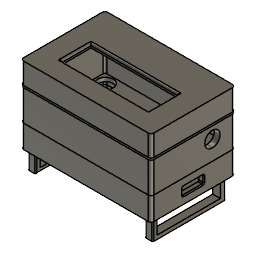
Irfan Hazlan - Device Case CAD Model (Autodesk Fusion 360 archive; units mm, degrees)
design "Irfan Hazlan - Device Case CAD Model" references "Prototype"
part number: 2026-02-20-13-36-55-425
Autodesk Fusion 360 part; units mm, degrees
derive "Sketch1"
sketch "sketch 219" plane through (0, 0, 0) normal (0, 0, 1) x (1, 0, 0)
  line L0 (1.5, 0) -> (66.5, 0)
  line L1 (68, 1.5) -> (68, 42.5)
  line L2 (66.5, 44) -> (1.5, 44)
  line L3 (0, 42.5) -> (0, 1.5)
  arc A0 (1.5, 44) -> (0, 42.5) centre (1.5, 42.5) ccw
  arc A1 (68, 42.5) -> (66.5, 44) centre (66.5, 42.5) ccw
  arc A2 (66.5, 0) -> (68, 1.5) centre (66.5, 1.5) ccw
  arc A3 (0, 1.5) -> (1.5, 0) centre (1.5, 1.5) ccw
  line L4 (2, 41) -> (2, 3)
  line L5 (3, 2) -> (65, 2)
  line L6 (66, 3) -> (66, 41)
  line L7 (65, 42) -> (3, 42)
  line L8 (4, 3) -> (64, 3)
  line L9 (65, 4) -> (65, 40)
  line L10 (64, 41) -> (4, 41)
  line L11 (3, 40) -> (3, 4)
  arc A4 (3, 42) -> (2, 41) centre (3, 41) ccw
  arc A5 (2, 3) -> (3, 2) centre (3, 3) ccw
  arc A6 (65, 2) -> (66, 3) centre (65, 3) ccw
  arc A7 (66, 41) -> (65, 42) centre (65, 41) ccw
  arc A8 (65, 40) -> (64, 41) centre (64, 40) ccw
  arc A9 (4, 41) -> (3, 40) centre (4, 40) ccw
  arc A10 (3, 4) -> (4, 3) centre (4, 4) ccw
  arc A11 (64, 3) -> (65, 4) centre (64, 4) ccw
  arc A12 (164, 3) -> (165, 4) centre (164, 4) ccw
  arc A13 (101.5, 44) -> (100, 42.5) centre (101.5, 42.5) ccw
  arc A14 (100, 1.5) -> (101.5, 0) centre (101.5, 1.5) ccw
  arc A15 (165, 2) -> (166, 3) centre (165, 3) ccw
  line L12 (166, 3) -> (166, 41)
  line L13 (103, 40) -> (103, 4)
  line L14 (165, 42) -> (103, 42)
  line L15 (103, 2) -> (165, 2)
  arc A16 (102, 3) -> (103, 2) centre (103, 3) ccw
  arc A17 (166.5, 0) -> (168, 1.5) centre (166.5, 1.5) ccw
  arc A18 (165, 40) -> (164, 41) centre (164, 40) ccw
  arc A19 (103, 42) -> (102, 41) centre (103, 41) ccw
  arc A20 (166, 41) -> (165, 42) centre (165, 41) ccw
  line L16 (166.5, 44) -> (101.5, 44)
  line L17 (101.5, 0) -> (166.5, 0)
  line L18 (168, 1.5) -> (168, 42.5)
  line L19 (102, 41) -> (102, 3)
  arc A21 (168, 42.5) -> (166.5, 44) centre (166.5, 42.5) ccw
  line L20 (100, 42.5) -> (100, 1.5)
  line L21 (104, 3) -> (164, 3)
  arc A22 (103, 4) -> (104, 3) centre (104, 4) ccw
  line L22 (165, 4) -> (165, 40)
  arc A23 (104, 41) -> (103, 40) centre (104, 40) ccw
  line L23 (164, 41) -> (104, 41)
  arc A24 (264, 3) -> (265, 4) centre (264, 4) ccw
  arc A25 (201.5, 44) -> (200, 42.5) centre (201.5, 42.5) ccw
  arc A26 (200, 1.5) -> (201.5, 0) centre (201.5, 1.5) ccw
  arc A27 (265, 2) -> (266, 3) centre (265, 3) ccw
  line L24 (266, 3) -> (266, 41)
  line L25 (203, 40) -> (203, 4)
  line L26 (265, 42) -> (203, 42)
  line L27 (203, 2) -> (265, 2)
  arc A28 (202, 3) -> (203, 2) centre (203, 3) ccw
  arc A29 (266.5, 0) -> (268, 1.5) centre (266.5, 1.5) ccw
  arc A30 (265, 40) -> (264, 41) centre (264, 40) ccw
  arc A31 (203, 42) -> (202, 41) centre (203, 41) ccw
  arc A32 (266, 41) -> (265, 42) centre (265, 41) ccw
  line L28 (266.5, 44) -> (201.5, 44)
  line L29 (201.5, 0) -> (266.5, 0)
  line L30 (268, 1.5) -> (268, 42.5)
  line L31 (202, 41) -> (202, 3)
  arc A33 (268, 42.5) -> (266.5, 44) centre (266.5, 42.5) ccw
  line L32 (200, 42.5) -> (200, 1.5)
  line L33 (204, 3) -> (264, 3)
  arc A34 (203, 4) -> (204, 3) centre (204, 4) ccw
  line L34 (265, 4) -> (265, 40)
  arc A35 (204, 41) -> (203, 40) centre (204, 40) ccw
  line L35 (264, 41) -> (204, 41)
  point P0 (68, 0)
  point P1 (0, 44)
  point P2 (100, 44)
  point P3 (168, 0)
  point P4 (100, 0)
  point P5 (100, 0)
  point P6 (200, 44)
  point P7 (268, 0)
  point P8 (200, 0)
  point P9 (200, 0)
extrude "Extrude1" add sketch "sketch 219" along normal blind 2 contours L8 L9 L10 L11 A8 A9 A10 A11 makes body 1
extrude "Extrude2" add sketch "sketch 219" along normal blind 10 contours L4 L5 L6 L7 A4 A5 A6 A7 bodies 1
extrude "Extrude3" add sketch "sketch 219" along normal blind 12 contours L0 L1 L2 L3 A0 A1 A2 A3 bodies 1
extrude "Extrude4" add sketch "sketch 219" along normal blind 20 separate body contours A15 L12 L14 L15 A16 A19 A20 L19 makes body 2
extrude "Extrude5" add sketch "sketch 219" along normal blind 2 from surface at 10 contours A12 L13 A18 L21 A22 L22 A23 L23 bodies 2
extrude "Extrude6" add sketch "sketch 219" along normal blind 16 from surface at 2 contours A13 A14 A17 L16 L17 L18 A21 L20 bodies 2
move_face "MoveFace1" by (0, 0, -6) 1 faces at (144, 28.3333, 12) on bodies 2
extrude "Extrude7" add sketch "sketch 219" along normal blind 12 contours A12 L13 A18 L21 A22 L22 A23 L23 bodies 2
sketch "Sketch1" plane through (0, 0, 12) normal (0, 0, 1) x (-1, 0, 0)
  line L0 (-164, -41) -> (-104, -41)
  arc A0 (-104, -41) -> (-103, -40) centre (-104, -40) ccw
  line L1 (-103, -40) -> (-103, -4)
  arc A1 (-103, -4) -> (-104, -3) centre (-104, -4) ccw
  line L2 (-104, -3) -> (-164, -3)
  arc A2 (-164, -3) -> (-165, -4) centre (-164, -4) ccw
  line L3 (-165, -4) -> (-165, -40)
  arc A3 (-165, -40) -> (-164, -41) centre (-164, -40) ccw
  circle A4 centre (-108.0439, -36.228) radius 2.5
  circle A5 centre (-108.0439, -36.228) radius 4
  dimension "d17" = 5
  dimension "d114" = 8
  constraint concentric A4 A5
  measures "d17" diameter of A4
  measures "d114" diameter of A5
extrude "Extrude8" cut sketch "Sketch1" against normal blind 2 contours A4 bodies 2
copy_body "CopyPasteBodies3" bodies 1 makes body 3
move_body "Move2" bodies 3 to x (1, 0, 0) y (0, 1, 0) z (0, 0, 1) at (200, 0, 0)
move_body "Move3" bodies 3 to x (1, 0, 0) y (0, 1, 0) z (0, 0, 1) at (0, 0, 10)
move_body "Move4" bodies 3 to x (-1, 0, 0) y (0, 1, 0) z (0, 0, -1) at (536, 0, 20)
move_body "Move5" bodies 3 to x (1, 0, 0) y (0, 1, 0) z (0, 0, 1) at (-70, 0, 0)
sketch "Sketch2" plane through (0, 0, 10) normal (0, 0, 1) x (-1, 0, 0)
  arc A0 (-264.5, 0) -> (-266, -1.5) centre (-264.5, -1.5) ccw
  line L0 (-266, -1.5) -> (-266, -42.5)
  arc A1 (-266, -42.5) -> (-264.5, -44) centre (-264.5, -42.5) ccw
  line L1 (-264.5, -44) -> (-199.5, -44)
  arc A2 (-199.5, -44) -> (-198, -42.5) centre (-199.5, -42.5) ccw
  line L2 (-198, -42.5) -> (-198, -1.5)
  arc A3 (-198, -1.5) -> (-199.5, 0) centre (-199.5, -1.5) ccw
  line L3 (-199.5, 0) -> (-264.5, 0)
  line L4 (-209.1663, -25.5187) -> (-254.1663, -25.5187)
  line L5 (-254.1663, -25.5187) -> (-254.1663, -10.5187)
  line L6 (-254.1663, -10.5187) -> (-209.1663, -10.5187)
  line L7 (-209.1663, -10.5187) -> (-209.1663, -25.5187)
  dimension "d30" = 45
  dimension "d31" = 15
  constraint horizontal L4
  constraint vertical L5
  constraint horizontal L6
  constraint vertical L7
  measures "d30" distance of L4.start L4.end
  measures "d31" distance of L4.end L5.end
extrude "Extrude9" cut sketch "Sketch2" against normal blind 2 contours L4 L5 L6 L7 bodies 3
fillet "Fillet1" radius 1 2 edges at (254.1663, 18.0187, 10) (231.6663, 25.5187, 10) on bodies 3
fillet "Fillet2" radius 1 2 edges at (232.1663, 10.5187, 10) (209.1663, 18.5187, 10) on bodies 3
sketch "Sketch3" plane through (0, 0, 0) normal (0, 0, -1) x (1, 0, 0)
  arc A0 (1.5, 0) -> (0, -1.5) centre (1.5, -1.5) ccw
  line L0 (0, -1.5) -> (0, -42.5)
  arc A1 (0, -42.5) -> (1.5, -44) centre (1.5, -42.5) ccw
  line L1 (1.5, -44) -> (66.5, -44)
  arc A2 (66.5, -44) -> (68, -42.5) centre (66.5, -42.5) ccw
  line L2 (68, -42.5) -> (68, -1.5)
  arc A3 (68, -1.5) -> (66.5, 0) centre (66.5, -1.5) ccw
  line L3 (66.5, 0) -> (1.5, 0)
  line L4 (66.9452, -39.9907) -> (62.9452, -39.9907)
  line L5 (62.9452, -39.9907) -> (62.9452, -1.9907)
  line L6 (62.9452, -1.9907) -> (66.9452, -1.9907)
  line L7 (66.9452, -1.9907) -> (66.9452, -39.9907)
  line L8 (5.9452, -1.9907) -> (5.9452, -39.9907)
  line L9 (5.9452, -39.9907) -> (1.9452, -39.9907)
  line L10 (1.9452, -39.9907) -> (1.9452, -1.9907)
  line L11 (1.9452, -1.9907) -> (5.9452, -1.9907)
  dimension "d38" = 38
  dimension "d39" = 4
  dimension "d40" = 38
  dimension "d41" = 4
  constraint horizontal L4
  constraint vertical L5
  constraint horizontal L6
  constraint vertical L7
  constraint horizontal L9
  constraint vertical L10
  constraint horizontal L11
  constraint vertical L8
  measures "d38" distance of L4.end L5.end
  measures "d39" distance of L4.start L4.end
  measures "d40" distance of L10.end L9.end
  measures "d41" distance of L8.end L9.end
extrude "Extrude10" add sketch "Sketch3" along normal blind 10 contours L4 L5 L6 L7 bodies 1
extrude "Extrude11" add sketch "Sketch3" along normal blind 10 contours L8 L9 L10 L11 bodies 1
sketch "Sketch4" plane through (1.9452, 0, 0) normal (-1, 0, 0) x (0, -1, 0)
  line L0 (-1.9907, 0) -> (-39.9907, 0)
  line L1 (-39.9907, 0) -> (-39.9907, -10)
  line L2 (-39.9907, -10) -> (-1.9907, -10)
  line L3 (-1.9907, -10) -> (-1.9907, 0)
  line L4 (-37.2414, 0.0076) -> (-4.2414, 0.0076)
  line L5 (-4.2414, 0.0076) -> (-4.2414, -7.9924)
  line L6 (-4.2414, -7.9924) -> (-37.2414, -7.9924)
  line L7 (-37.2414, -7.9924) -> (-37.2414, 0.0076)
  line L8 (-37.2414, -7.9924, -61) -> (-37.2414, 0.0076, -61)
  line L9 (-4.2414, -7.9924, -61) -> (-37.2414, -7.9924, -61)
  line L10 (-4.2414, 0.0076, -61) -> (-4.2414, -7.9924, -61)
  line L11 (-37.2414, 0.0076, -61) -> (-4.2414, 0.0076, -61)
  dimension "d46" = 8
  dimension "d47" = 33
  dimension "d49" = 33
  constraint horizontal L4
  constraint vertical L5
  constraint horizontal L6
  constraint vertical L7
  measures "d46" distance of L4.start L6.end
  measures "d47" distance of L4.start L4.end
  measures "d49" distance of L4.start L4.end
extrude "Extrude12" cut sketch "Sketch4" against normal blind 4 contours L8 L9 L10 L11 in plane through (62.9452, 0, 0) normal (-1, 0, 0) bodies 1
extrude "Extrude13" cut sketch "Sketch4" against normal blind 4 contours L0 L5 L6 L7 | L0 L4 L5 L7 bodies 1
sketch "Sketch5" plane through (0, 2, 0) normal (0, -1, 0) x (1, 0, 0)
  line L0 (165, 2) -> (103, 2)
  line L1 (103, 2) -> (103, 0)
  line L2 (103, 0) -> (165, 0)
  line L3 (165, 0) -> (165, 2)
  line L4 (103, 1) -> (134, 1)
  line L5 (103, 2) -> (134, 0)
  line L6 (103, 0) -> (134, 2)
  line L7 (121, 0.375) -> (116, 0.375)
  line L8 (116, 0.375) -> (116, 1.625)
  line L9 (116, 1.625) -> (121, 1.625)
  line L10 (121, 1.625) -> (121, 0.375)
  line L11 (121, 0.375) -> (116, 1.625) construction
  line L12 (116, 0.375) -> (121, 1.625) construction
  line L13 (134, 2) -> (134, 0)
  line L14 (152, 0.375) -> (152, 1.625)
  line L15 (152, 1.625) -> (147, 1.625)
  line L16 (147, 0.375) -> (152, 0.375)
  line L17 (147, 1.625) -> (147, 0.375)
  point P0 (118.5, 1)
  dimension "d54" = 31
  dimension "d55" = 5
  dimension "d56" = 1.25
  constraint midpoint L1 L4.start
  constraint perpendicular L1 L4
  constraint coincident L0.end L1.start
  constraint midpoint L2 L5.end
  constraint coincident L1.end L2.start
  constraint midpoint L0 L6.end
  constraint horizontal L7
  constraint perpendicular L7 L8
  constraint parallel L7 L9
  constraint parallel L8 L10
  constraint coincident L11 P0
  constraint coincident L12 P0
  constraint midpoint L5 P0
  constraint symmetric L7.start L13 L16.start
  constraint symmetric L7.end L13 L14.start
  constraint symmetric L8.end L13 L14.end
  constraint symmetric L9.end L13 L15.end
  measures "d54" distance of L4.start L4.end
  measures "d55" distance of L8.end L9.end
  measures "d56" distance of L7.end L8.end
sketch "Sketch6" plane through (0, 2, 0) normal (0, -1, 0) x (1, 0, 0)
sketch "Sketch7" plane through (0, 42, 0) normal (0, 1, 0) x (-1, 0, 0)
  line L0 (-103, 2) -> (-165, 2)
  line L1 (-165, 2) -> (-165, 0)
  line L2 (-165, 0) -> (-103, 0)
  line L3 (-103, 0) -> (-103, 2)
  line L4 (-147, 0.375) -> (-152, 0.375)
  line L5 (-147, 1.625) -> (-147, 0.375)
  line L6 (-152, 1.625) -> (-147, 1.625)
  line L7 (-152, 0.375) -> (-152, 1.625)
  line L8 (-116, 1.625) -> (-121, 1.625)
  line L9 (-121, 0.375) -> (-116, 0.375)
  line L10 (-116, 0.375) -> (-116, 1.625)
  line L11 (-121, 1.625) -> (-121, 0.375)
sketch "Sketch8" plane through (0, 0, -2) normal (0, 0, -1) x (1, 0, 0)
  arc A0 (200, -41) -> (201, -42) centre (201, -41) ccw
  line L0 (200, -41) -> (200, -3)
  arc A1 (201, -2) -> (200, -3) centre (201, -3) ccw
  line L1 (201, -2) -> (263, -2)
  arc A2 (264, -3) -> (263, -2) centre (263, -3) ccw
  line L2 (264, -3) -> (264, -41)
  arc A3 (263, -42) -> (264, -41) centre (263, -41) ccw
  line L3 (263, -42) -> (201, -42)
  arc A4 (266, -1.5) -> (264.5, 0) centre (264.5, -1.5) ccw
  line L4 (264.5, 0) -> (199.5, 0)
  arc A5 (199.5, 0) -> (198, -1.5) centre (199.5, -1.5) ccw
  line L5 (198, -1.5) -> (198, -42.5)
  arc A6 (198, -42.5) -> (199.5, -44) centre (199.5, -42.5) ccw
  line L6 (199.5, -44) -> (264.5, -44)
  arc A7 (264.5, -44) -> (266, -42.5) centre (264.5, -42.5) ccw
  line L7 (266, -42.5) -> (266, -1.5)
extrude "Extrude14" add sketch "Sketch7" along normal blind 1 draft -50 contours L4 L5 L6 L7 | L8 L9 L10 L11 bodies 2
extrude "Extrude15" add sketch "Sketch5" along normal blind 1 draft -50 contours L14 L15 L16 L17 bodies 2
extrude "Extrude16" add sketch "Sketch5" along normal blind 1 draft -50 contours L4 L6 L10 | L5 L6 L8 L9 L10 | L4 L5 L8 | L4 L6 L8 | L4 L5 L10 | L5 L6 L7 L8 L10 bodies 2
sketch "Sketch12" plane through (0, 0, 0) normal (0, -1, 0) x (1, 0, 0)
  line L0 (101.5, 2) -> (166.5, 2)
  line L1 (166.5, 2) -> (166.5, 18)
  line L2 (166.5, 18) -> (101.5, 18)
  line L3 (101.5, 18) -> (101.5, 2)
  line L4 (105.009, 18) -> (105.009, 9)
  line L5 (101.5, 9.1208) -> (166.5, 9.1208)
  dimension "d66" = 9
  dimension "d67" = 65
  constraint coincident L2 L4.start
  constraint perpendicular L2 L4
  constraint coincident L3 L5.start
  constraint perpendicular L3 L5
  measures "d66" distance of L4.start L4.end
  measures "d67" distance of L5.start L5.end
sketch "Sketch13" plane through (0, 2, 0) normal (0, -1, 0) x (1, 0, 0)
  line L0 (103, 18) -> (165, 18)
  line L1 (165, 18) -> (165, 20)
  line L2 (165, 20) -> (103, 20)
  line L3 (103, 20) -> (103, 18)
  line L4 (116, 1.625) -> (121, 1.625)
  line L5 (116, 0.375) -> (116, 1.625)
  line L6 (121, 0.375) -> (116, 0.375)
  line L7 (121, 1.625) -> (121, 0.375)
  line L8 (152, 1.625) -> (147, 1.625)
  line L9 (147, 1.625) -> (147, 0.375)
  line L10 (147, 0.375) -> (152, 0.375)
  line L11 (152, 0.375) -> (152, 1.625)
sketch "Sketch14" plane through (0, 2, 0) normal (0, -1, 0) x (1, 0, 0)
  line L0 (134.0523, 17.9964) -> (134.0523, 19.9964)
  line L1 (103.1583, 20.0029) -> (134.0523, 17.9964)
  line L2 (103.1583, 17.9964) -> (134.2435, 20.0029)
  line L3 (121.1529, 18.3716) -> (116.1529, 18.3716)
  line L4 (116.1529, 18.3716) -> (116.1529, 19.6216)
  line L5 (116.1529, 19.6216) -> (121.1529, 19.6216)
  line L6 (121.1529, 19.6216) -> (121.1529, 18.3716)
  line L7 (121.1529, 18.3716) -> (116.1529, 19.6216) construction
  line L8 (116.1529, 18.3716) -> (121.1529, 19.6216) construction
  line L9 (151.9517, 19.6216) -> (146.9517, 19.6216)
  line L10 (151.9517, 18.3716) -> (151.9517, 19.6216)
  line L11 (146.9517, 18.3716) -> (151.9517, 18.3716)
  line L12 (146.9517, 19.6216) -> (146.9517, 18.3716)
  point P0 (118.6529, 18.9966)
  dimension "d68" = 2
  dimension "d69" = 5
  dimension "d70" = 1.25
  constraint vertical L0
  constraint horizontal L3
  constraint perpendicular L3 L4
  constraint parallel L3 L5
  constraint parallel L4 L6
  constraint coincident L7 P0
  constraint coincident L8 P0
  constraint coincident L1 P0
  constraint coincident L2 P0
  constraint symmetric L0 L3.start L11.start
  constraint symmetric L0 L3.end L10.start
  constraint symmetric L0 L4.end L9.start
  constraint symmetric L0 L5.end L9.end
  measures "d68" distance of L0.start L0.end
  measures "d69" distance of L4.end L5.end
  measures "d70" distance of L3.end L4.end
sketch "Sketch15" plane through (0, 2, 0) normal (0, -1, 0) x (1, 0, 0)
  line L0 (116.1529, 19.6216) -> (121.1529, 19.6216)
  line L1 (116.1529, 18.3716) -> (116.1529, 19.6216)
  line L2 (121.1529, 18.3716) -> (116.1529, 18.3716)
  line L3 (121.1529, 19.6216) -> (121.1529, 18.3716)
  line L4 (146.9517, 19.6216) -> (146.9517, 18.3716)
  line L5 (151.9517, 19.6216) -> (146.9517, 19.6216)
  line L6 (146.9517, 18.3716) -> (151.9517, 18.3716)
  line L7 (151.9517, 18.3716) -> (151.9517, 19.6216)
extrude "Extrude18" add sketch "Sketch14" along normal blind 1 draft -50 contours L9 L10 L11 L12 bodies 2
sketch "Sketch16" plane through (0, 42, 0) normal (0, 1, 0) x (-1, 0, 0)
  line L0 (-165, 18) -> (-103, 18)
  line L1 (-103, 18) -> (-103, 20)
  line L2 (-103, 20) -> (-165, 20)
  line L3 (-165, 20) -> (-165, 18)
  line L4 (-116.1496, 18.3709) -> (-121.1496, 18.3709)
  line L5 (-121.1496, 18.3709) -> (-121.1496, 19.6209)
  line L6 (-121.1496, 19.6209) -> (-116.1496, 19.6209)
  line L7 (-116.1496, 19.6209) -> (-116.1496, 18.3709)
  line L8 (-116.1496, 18.3709) -> (-121.1496, 19.6209) construction
  line L9 (-121.1496, 18.3709) -> (-116.1496, 19.6209) construction
  line L10 (-134.0576, 20) -> (-134.0576, 18)
  line L11 (-134.0576, 20) -> (-165, 20)
  line L12 (-146.9656, 19.6209) -> (-151.9656, 19.6209)
  line L13 (-146.9656, 18.3709) -> (-146.9656, 19.6209)
  line L14 (-151.9656, 18.3709) -> (-146.9656, 18.3709)
  line L15 (-151.9656, 19.6209) -> (-151.9656, 18.3709)
  point P0 (-118.6496, 18.9959)
  dimension "d75" = 5
  dimension "d76" = 1.25
  constraint horizontal L4
  constraint perpendicular L4 L5
  constraint parallel L4 L6
  constraint parallel L5 L7
  constraint coincident L8 P0
  constraint coincident L9 P0
  constraint coincident L2 L10.start
  constraint coincident L0 L10.end
  constraint perpendicular L0 L10
  constraint coincident L2.end L3.start
  constraint symmetric L4.start L10 L14.start
  constraint symmetric L4.end L10 L13.start
  constraint symmetric L5.end L10 L12.start
  constraint symmetric L6.end L10 L12.end
  measures "d75" distance of L5.end L6.end
  measures "d76" distance of L4.end L5.end
sketch "Sketch17" plane through (0, 42, 0) normal (0, 1, 0) x (-1, 0, 0)
  line L0 (-165, 18) -> (-103, 18)
  line L1 (-103, 18) -> (-103, 20)
  line L2 (-103, 20) -> (-165, 20)
  line L3 (-165, 20) -> (-165, 18)
  line L4 (-121.1488, 19.6218) -> (-116.1488, 19.6218)
  line L5 (-116.1488, 19.6218) -> (-116.1488, 18.3718)
  line L6 (-116.1488, 18.3718) -> (-121.1488, 18.3718)
  line L7 (-121.1488, 18.3718) -> (-121.1488, 19.6218)
  line L8 (-151.9516, 19.6215) -> (-146.9516, 19.6215)
  line L9 (-146.9516, 19.6215) -> (-146.9516, 18.3715)
  line L10 (-146.9516, 18.3715) -> (-151.9516, 18.3715)
  line L11 (-151.9516, 18.3715) -> (-151.9516, 19.6215)
  dimension "d83" = 5
  dimension "d84" = 1.25
  dimension "d85" = 5
  dimension "d86" = 1.25
  constraint horizontal L4
  constraint vertical L5
  constraint horizontal L6
  constraint vertical L7
  constraint horizontal L8
  constraint vertical L9
  constraint horizontal L10
  constraint vertical L11
  measures "d83" distance of L4.start L4.end
  measures "d84" distance of L4.end L5.end
  measures "d85" distance of L8.start L8.end
  measures "d86" distance of L8.end L9.end
extrude "Extrude22" add sketch "Sketch17" along normal blind 1 draft -50 contours L8 L9 L10 L11 bodies 2
sketch "Sketch18" plane through (0, 42, 0) normal (0, 1, 0) x (-1, 0, 0)
  line L0 (-151.9516, 18.3715) -> (-151.9516, 19.6215)
  line L1 (-151.9516, 19.6215) -> (-146.9516, 19.6215)
  line L2 (-146.9516, 19.6215) -> (-146.9516, 18.3715)
  line L3 (-146.9516, 18.3715) -> (-151.9516, 18.3715)
  line L4 (-165, 18) -> (-103, 18)
  line L5 (-103, 18) -> (-103, 20)
  line L6 (-103, 20) -> (-165, 20)
  line L7 (-165, 20) -> (-165, 18)
  line L8 (-121.1526, 19.6212) -> (-116.1526, 19.6212)
  line L9 (-116.1526, 19.6212) -> (-116.1526, 18.3712)
  line L10 (-116.1526, 18.3712) -> (-121.1526, 18.3712)
  line L11 (-121.1526, 18.3712) -> (-121.1526, 19.6212)
  dimension "d91" = 5
  dimension "d92" = 1.25
  constraint horizontal L8
  constraint vertical L9
  constraint horizontal L10
  constraint vertical L11
  measures "d91" distance of L8.start L8.end
  measures "d92" distance of L8.end L9.end
extrude "Extrude24" add sketch "Sketch18" along normal blind 1 draft -50 contours L8 L9 L10 L11 bodies 2
extrude "Extrude25" add sketch "Sketch14" along normal blind 1 draft -50 contours L1 L2 L3 L4 L6 | L1 L2 L6 | L1 L2 L4 L5 L6 | L1 L2 L4 bodies 2
sketch "Sketch19" plane through (0, 42, 0) normal (0, -1, 0) x (1, 0, 0)
  line L0 (3, 10) -> (65, 10)
  line L1 (65, 10) -> (65, 12)
  line L2 (65, 12) -> (3, 12)
  line L3 (3, 12) -> (3, 10)
  line L4 (3, 12) -> (34, 10)
  line L5 (3, 10) -> (34, 12)
  line L6 (21.1, 11.675) -> (15.9, 11.675)
  line L7 (15.9, 11.675) -> (15.9, 10.325)
  line L8 (15.9, 10.325) -> (21.1, 10.325)
  line L9 (21.1, 10.325) -> (21.1, 11.675)
  line L10 (21.1, 11.675) -> (15.9, 10.325) construction
  line L11 (15.9, 11.675) -> (21.1, 10.325) construction
  line L12 (34.05, 12) -> (34.05, 10)
  line L13 (47, 11.675) -> (52.2, 11.675)
  line L14 (47, 10.325) -> (47, 11.675)
  line L15 (52.2, 10.325) -> (47, 10.325)
  line L16 (52.2, 11.675) -> (52.2, 10.325)
  point P0 (18.5, 11)
  dimension "d97" = 5.2
  dimension "d98" = 1.35
  constraint coincident L2.end L3.start
  constraint midpoint L0 L4.end
  constraint coincident L0.start L3.end
  constraint midpoint L2 L5.end
  constraint horizontal L6
  constraint perpendicular L6 L7
  constraint parallel L6 L8
  constraint parallel L7 L9
  constraint coincident L10 P0
  constraint coincident L11 P0
  constraint coincident L4 P0
  constraint coincident L2 L12.start
  constraint coincident L0 L12.end
  constraint perpendicular L0 L12
  constraint symmetric L6.start L12 L13.start
  constraint symmetric L6.end L12 L13.end
  constraint symmetric L7.end L12 L15.start
  constraint symmetric L8.end L12 L14.start
  constraint midpoint L4 P0
  measures "d97" distance of L7.end L8.end
  measures "d98" distance of L6.start L8.end
sketch "Sketch20" plane through (0, 2, 0) normal (0, 1, 0) x (-1, 0, 0)
  line L0 (-65, 10) -> (-3, 10)
  line L1 (-3, 10) -> (-3, 12)
  line L2 (-3, 12) -> (-65, 12)
  line L3 (-65, 12) -> (-65, 10)
  line L4 (-21.1, 11.675) -> (-15.9, 11.675)
  line L5 (-15.9, 11.675) -> (-15.9, 10.325)
  line L6 (-15.9, 10.325) -> (-21.1, 10.325)
  line L7 (-21.1, 10.325) -> (-21.1, 11.675)
  line L8 (-52.2, 11.675) -> (-52.2, 10.325)
  line L9 (-47, 11.675) -> (-52.2, 11.675)
  line L10 (-47, 10.325) -> (-47, 11.675)
  line L11 (-52.2, 10.325) -> (-47, 10.325)
extrude "Extrude26" cut sketch "Sketch20" against normal blind 1 draft -50 contours L4 L5 L6 L7 | L8 L9 L10 L11 bodies 1
extrude "Extrude27" cut sketch "Sketch19" against normal blind 1 draft -50 contours L4 L5 L7 | L4 L5 L7 L8 L9 | L4 L5 L9 | L4 L5 L6 L7 L9 | L13 L14 L15 L16 bodies 1
sketch "Sketch21" plane through (0, 2, 0) normal (0, 1, 0) x (-1, 0, 0)
  line L0 (-201, 0) -> (-263, 0)
  line L1 (-263, 0) -> (-263, -2)
  line L2 (-263, -2) -> (-201, -2)
  line L3 (-201, -2) -> (-201, 0)
  line L4 (-201, 0) -> (-232, 0)
  line L5 (-232, 0) -> (-232, -2)
  line L6 (-232, -2) -> (-201, 0)
  line L7 (-201, -2) -> (-232, 0)
  line L8 (-214, -0.675) -> (-219, -0.675)
  line L9 (-219, -0.675) -> (-219, 0.675)
  line L10 (-219, 0.675) -> (-214, 0.675)
  line L11 (-214, 0.675) -> (-214, -0.675)
  line L12 (-214, -0.675) -> (-219, 0.675) construction
  line L13 (-219, -0.675) -> (-214, 0.675) construction
  line L14 (-250, -0.675) -> (-245, -0.675)
  line L15 (-250, 0.675) -> (-250, -0.675)
  line L16 (-245, 0.675) -> (-250, 0.675)
  line L17 (-245, -0.675) -> (-245, 0.675)
  point P0 (-216.5, -1)
  dimension "d103" = 5
  dimension "d104" = 1.35
  constraint coincident L0.start L3.end
  constraint coincident L2.end L3.start
  measures "d103" distance of L9.end L10.end
  measures "d104" distance of L8.end L9.end
sketch "Sketch22" plane through (0, 42, 0) normal (0, -1, 0) x (1, 0, 0)
  line L0 (263, 0) -> (201, 0)
  line L1 (201, 0) -> (201, -2)
  line L2 (201, -2) -> (263, -2)
  line L3 (263, -2) -> (263, 0)
  line L4 (245, -0.675) -> (245, 0.675)
  line L5 (250, -0.675) -> (245, -0.675)
  line L6 (245, 0.675) -> (250, 0.675)
  line L7 (250, 0.675) -> (250, -0.675)
  line L8 (214, -0.675) -> (219, -0.675)
  line L9 (219, -0.675) -> (219, 0.675)
  line L10 (219, 0.675) -> (214, 0.675)
  line L11 (214, 0.675) -> (214, -0.675)
extrude "Extrude28" cut sketch "Sketch21" against normal blind 1 draft -50 contours L0 L4 L8 L9 L11 | L0 L4 L9 L10 L11 | L0 L14 L15 L17 | L0 L15 L16 L17 bodies 3
extrude "Extrude29" cut sketch "Sketch22" against normal blind 1 draft -50 contours L0 L4 L5 L7 | L0 L4 L6 L7 | L0 L8 L9 L11 | L0 L9 L10 L11 bodies 3
extrude "Extrude31" cut sketch "sketch 219" along normal blind 10 contours A12 L13 A18 L21 A22 L22 A23 L23 bodies 2
extrude "Extrude32" cut sketch "Sketch1" against normal blind 2 contours A4 | A5 bodies 2
move_face "MoveFace4" to x (1, 0, 0) y (0, 1, 0) z (0, 0, 1) at (0, 0, -7) 3 faces at (146.5493, 26.1642, 10) (146.5493, 26.1642, 12) (104.0638, 36.6263, 11.3333) on bodies 2
sketch "Sketch25" plane through (103, 0, 0) normal (1, 0, 0) x (0, 1, 0)
  line L0 (4, 5) -> (40, 5)
  line L1 (40, 5) -> (40, 20)
  line L2 (40, 20) -> (4, 20)
  line L3 (4, 20) -> (4, 5)
  line L4 (40, 20) -> (40, 12)
  line L5 (40, 12) -> (4, 12)
  line L6 (42.5, 2, -3) -> (1.5, 2, -3)
  line L7 (1.5, 2, -3) -> (1.5, 18, -3)
  line L8 (1.5, 18, -3) -> (42.5, 18, -3)
  line L9 (42.5, 18, -3) -> (42.5, 2, -3)
  line L10 (4, 10, -3) -> (40, 10, -3)
  line L11 (21.95, 12) -> (21.95, 10)
  line L12 (22.45, 10.5131) -> (21.45, 10.5131)
  line L13 (21.45, 10.5131) -> (21.45, 9.5131)
  line L14 (21.45, 9.5131) -> (22.45, 9.5131)
  line L15 (22.45, 9.5131) -> (22.45, 10.5131)
  line L16 (22.45, 10.5131) -> (21.45, 9.5131) construction
  line L17 (21.45, 10.5131) -> (22.45, 9.5131) construction
  line L18 (22.45, 10.5131) -> (6.45, 10.5131)
  line L19 (6.45, 10.5131) -> (6.45, 8.5131)
  line L20 (6.45, 8.5131) -> (22.45, 8.5131)
  line L21 (22.45, 8.5131) -> (22.45, 10.5131)
  point P0 (22, 10)
  point P1 (21.95, 10.0131)
  dimension "d120" = 2
  dimension "d121" = 1
  dimension "d122" = 1
  dimension "d150" = 16
  dimension "d151" = 2
  constraint coincident L1.end L2.start
  constraint coincident L1 L4.end
  constraint coincident L3 L5.end
  constraint perpendicular L3 L5
  constraint coincident L5 L11.start
  constraint perpendicular L5 L11
  constraint horizontal L12
  constraint perpendicular L12 L13
  constraint parallel L12 L14
  constraint parallel L13 L15
  constraint coincident L16 P1
  constraint coincident L17 P1
  constraint coincident L11 P1
  constraint horizontal L18
  constraint vertical L19
  constraint horizontal L20
  constraint vertical L21
  measures "d120" distance of L11.start L11.end
  measures "d121" distance of L12.end L13.end
  measures "d122" distance of L13.end L14.end
  measures "d150" distance of L12.start L18.end
  measures "d151" distance of L12.start L20.end
sketch "Sketch26" plane through (165, 0, 0) normal (-1, 0, 0) x (0, -1, 0)
  line L0 (-40, 5) -> (-4, 5)
  line L1 (-4, 5) -> (-4, 20)
  line L2 (-4, 20) -> (-40, 20)
  line L3 (-40, 20) -> (-40, 5)
  line L4 (-22.45, 10.5131) -> (-21.45, 10.5131)
  line L5 (-21.45, 10.5131) -> (-21.45, 9.5131)
  line L6 (-22.45, 9.5131) -> (-22.45, 10.5131)
  line L7 (-21.45, 9.5131) -> (-22.45, 9.5131)
  line L8 (-22.45, 10.5131) -> (-6.45, 10.5131)
  line L9 (-6.45, 10.5131) -> (-6.45, 8.5131)
  line L10 (-6.45, 8.5131) -> (-22.45, 8.5131)
  line L11 (-22.45, 8.5131) -> (-22.45, 10.5131)
  dimension "d156" = 16
  dimension "d157" = 2
  constraint horizontal L8
  constraint vertical L9
  constraint horizontal L10
  constraint vertical L11
  constraint coincident L4.start L6.end
  measures "d156" distance of L4.start L8.end
  measures "d157" distance of L8.end L9.end
extrude "Extrude33" add sketch "Sketch25" along normal blind 2 contours L12 L13 L14 L15 L18 L21 bodies 2
extrude "Extrude34" add sketch "Sketch26" along normal blind 2 contours L4 L5 L6 L7 L8 L11 bodies 2
fillet "Fillet3" radius 0.5 5 edges at (62.9452, 39.9907, -5) (62.9452, 20.9907, -10) (66.9452, 39.9907, -5) (66.9452, 1.9907, -5) (62.9452, 1.9907, -5) on bodies 1
fillet "Fillet4" radius 0.5 6 edges at (5.9452, 1.9907, -5) (5.9452, 20.9907, -10) (1.9452, 1.9907, -5) (1.9452, 20.9907, -10) (1.9452, 39.9907, -5) (5.9452, 39.9907, -5) on bodies 1
sketch "Sketch27" plane through (65, 0, 0) normal (-1, 0, 0) x (0, -1, 0)
  line L0 (-40, 2) -> (-4, 2)
  line L1 (-4, 2) -> (-4, 10)
  line L2 (-4, 10) -> (-40, 10)
  line L3 (-40, 10) -> (-40, 2)
  line L4 (-40, 2) -> (-4, 10)
  line L5 (-40, 10) -> (-4, 2)
  line L6 (-27.5, 8) -> (-16.5, 8)
  line L7 (-16.5, 8) -> (-16.5, 4)
  line L8 (-16.5, 4) -> (-27.5, 4)
  line L9 (-27.5, 4) -> (-27.5, 8)
  line L10 (-27.5, 8) -> (-16.5, 4) construction
  line L11 (-16.5, 8) -> (-27.5, 4) construction
  line L12 (-40, 2) -> (-4, 2)
  line L13 (-4, 2) -> (-4, 10)
  line L14 (-4, 10) -> (-40, 10)
  line L15 (-40, 10) -> (-40, 2)
  point P0 (-22, 6)
  constraint coincident L0.start L3.end
  constraint coincident L1.end L2.start
  constraint coincident L2.end L3.start
  constraint coincident L0.end L1.start
  constraint horizontal L6
  constraint perpendicular L6 L7
  constraint parallel L6 L8
  constraint parallel L7 L9
  constraint coincident L10 P0
  constraint coincident L11 P0
  constraint midpoint L4 P0
sketch "Sketch28" plane through (3, 0, 0) normal (1, 0, 0) x (0, 1, 0)
  line L0 (4, 2) -> (40, 2)
  line L1 (40, 2) -> (40, 10)
  line L2 (40, 10) -> (4, 10)
  line L3 (4, 10) -> (4, 2)
  line L4 (16.5, 4) -> (27.5, 4)
  line L5 (16.5, 8) -> (16.5, 4)
  line L6 (27.5, 8) -> (16.5, 8)
  line L7 (27.5, 4) -> (27.5, 8)
extrude "Extrude39" add sketch "Sketch26" along normal blind 10 contours L4 L5 L6 L7 L8 L11 | L5 L7 L8 L9 L10 L11 bodies 2
extrude "Extrude35" cut sketch "Sketch27" against normal blind 5 contours L4 L5 L9 | L4 L5 L7 L8 L9 | L4 L5 L7 | L4 L5 L6 L7 L9 bodies 1
extrude "Extrude36" cut sketch "Sketch28" against normal blind 5 contours L4 L5 L6 L7 bodies 1
fillet "Fillet8" radius 0.5 4 faces at (66, 20.1667, 4) (66, 16.5, 6.6667) (66, 27.5, 5.3333) (66, 23.8333, 8) on bodies 1
fillet "Fillet9" radius 0.5 4 faces at (2, 16.5, 6.6667) (1, 23.8333, 4) (2, 27.5, 5.3333) (2, 23.8333, 8) on bodies 1
sketch "Sketch29" plane through (165, 0, 0) normal (-1, 0, 0) x (0, -1, 0)
  line L0 (-22.45, 8.5131) -> (-22.45, 10.5131)
  line L1 (-22.45, 10.5131) -> (-6.45, 10.5131)
  line L2 (-40, 5) -> (-4, 5)
  line L3 (-4, 5) -> (-4, 20)
  line L4 (-4, 20) -> (-40, 20)
  line L5 (-40, 20) -> (-40, 5)
  line L6 (-40, 5) -> (-40, 12)
  line L7 (-40, 12) -> (-32, 12)
  circle A0 centre (-32, 12) radius 4
  line L8 (-6.45, 10.5131) -> (-6.45, 8.5131)
  line L9 (-6.45, 8.5131) -> (-22.45, 8.5131)
  dimension "d145" = 8
  dimension "d146" = 8
  constraint coincident L2.start L5.end
  constraint coincident L5 L6.end
  constraint perpendicular L6 L7
  constraint coincident L7.end A0.centre
  measures "d145" distance of L6.end L7.end
  measures "d146" diameter of A0
extrude "Extrude37" cut sketch "Sketch29" against normal blind 5 contours A0 bodies 2
sketch "Sketch30" plane through (165, 0, 0) normal (-1, 0, 0) x (0, -1, 0)
  circle A0 centre (-32, 12) radius 4
  line L0 (-22.45, 8.5131) -> (-22.45, 10.5131)
  line L1 (-22.45, 10.5131) -> (-6.45, 10.5131)
  line L2 (-40, 5) -> (-4, 5)
  line L3 (-4, 5) -> (-4, 20)
  line L4 (-4, 20) -> (-40, 20)
  line L5 (-40, 20) -> (-40, 5)
  line L6 (-6.45, 10.5131) -> (-6.45, 8.5131)
  line L7 (-6.45, 8.5131) -> (-22.45, 8.5131)
extrude "Extrude38" add sketch "Sketch25" along normal blind 10 contours L12 L13 L14 L15 L18 L21 | L13 L14 L18 L19 L20 L21 bodies 2
fillet "Fillet10" radius 0.2 1 faces at (113, 11.7833, 9.1797) on bodies 2
sketch "Sketch23" plane through (0, 0, 5) normal (0, 0, 1) x (-1, 0, 0)
  line L0 (-164, -41) -> (-104, -41)
  arc A0 (-104, -41) -> (-103, -40) centre (-104, -40) ccw
  line L1 (-103, -40) -> (-103, -4)
  arc A1 (-103, -4) -> (-104, -3) centre (-104, -4) ccw
  line L2 (-104, -3) -> (-164, -3)
  arc A2 (-164, -3) -> (-165, -4) centre (-164, -4) ccw
  line L3 (-165, -4) -> (-165, -40)
  arc A3 (-165, -40) -> (-164, -41) centre (-164, -40) ccw
  circle A4 centre (-108.0439, -36.228) radius 4
sketch "Sketch24" plane through (0, 0, 0) normal (0, 0, -1) x (1, 0, 0)
  line L0 (102, -3) -> (102, -41)
  arc A0 (102, -41) -> (103, -42) centre (103, -41) ccw
  line L1 (103, -42) -> (165, -42)
  arc A1 (165, -42) -> (166, -41) centre (165, -41) ccw
  line L2 (166, -41) -> (166, -3)
  arc A2 (166, -3) -> (165, -2) centre (165, -3) ccw
  line L3 (165, -2) -> (103, -2)
  arc A3 (103, -2) -> (102, -3) centre (103, -3) ccw
  arc A4 (164, -41) -> (165, -40) centre (164, -40) ccw
  line L4 (164, -41) -> (104, -41)
  arc A5 (103, -40) -> (104, -41) centre (104, -40) ccw
  line L5 (103, -40) -> (103, -4)
  arc A6 (104, -3) -> (103, -4) centre (104, -4) ccw
  line L6 (104, -3) -> (164, -3)
  arc A7 (165, -4) -> (164, -3) centre (164, -4) ccw
  line L7 (165, -4) -> (165, -40)
extrude "Extrude42" cut 1 faces at (242.3333, 0.6667, -2) along direction (0, 0, 1) blind 1 on bodies 3 bodies 3
extrude "Extrude43" cut 1 faces at (238, 2.6667, 0) along direction (0, 0, 1) blind 1 on bodies 3 bodies 3
move_body "Move7" bodies 3 to x (1, 0, 0) y (0, 1, 0) z (0, 0, 1) at (-98, 0, 20)
move_body "Move8" bodies 1 to x (1, 0, 0) y (0, 1, 0) z (0, 0, 1) at (100, 0, -10)
move_body "Move10" [suppressed]
named bodies: "Bottom", "Bottom (1)", "Bottom (1) (1)"
